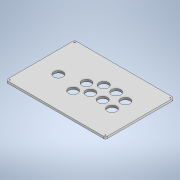
# Autodesk Inventor part: sega_straight
Saved by Autodesk Inventor 2022 (Build 260153000, 153)
## iProperties
Created: 2022-12-25
Part Number: sega_straight
Material: Generic
Document SubType Name: Modeling
Designer: Bunny
Density: 1 g/cm^3
Appearance: Default
Author: Bunny
Autodesk Inventor part; units mm, degrees
ref_plane "YZ Plane" through (0, 0, 0) normal (1, 0, 0) x (0, 1, 0)
ref_plane "XZ Plane" through (0, 0, 0) normal (0, 1, 0) x (-1, 0, 0)
ref_plane "XY Plane" through (0, 0, 0) normal (0, 0, 1) x (1, 0, 0)
sketch "Sketch1" plane through (0, 0, 0) normal (0, 1, 0) x (-1, 0, 0)
  line L0 (145, -100) -> (-145, -100)
  line L1 (-145, -100) -> (-145, 100)
  line L2 (-145, 100) -> (145, 100)
  line L3 (145, 100) -> (145, -100)
  line L4 (203, 0) -> (-203, 0) projected
  line L5 (0, -140) -> (0, 140) projected
  point P0 (0, 0)
  dimension "d30" = 290
  dimension "d31" = 200
  constraints: 8 end point, 2 parallel, 1 horizontal, 1 perpendicular, 2 other
  measures "d30" distance of L0.start L0.end
  measures "d31" distance of L0.end L1.end
extrude "Extrusion1" add sketch "Sketch1" along normal blind 6
sketch "Sketch2" plane through (0, 6, 0) normal (0, 1, 0) x (1, 0, 0)
  circle A0 centre (-19.75, -29.5) radius 13.5
  circle A1 centre (-82.75, -9.5) radius 13.5
  circle A2 centre (-19.75, 9.5) radius 13.5
  circle A3 centre (46.75, 29.5) radius 13.5
  circle A4 centre (82.75, 20.5) radius 13.5
  circle A5 centre (10.75, 29.5) radius 13.5
  circle A6 centre (10.75, -9.5) radius 13.5
  circle A7 centre (46.75, -9.5) radius 13.5
  circle A8 centre (82.75, -18.5) radius 13.5
  line L0 (-96.25, 43) -> (96.25, 43)
  line L1 (96.25, 43) -> (96.25, -43)
  line L2 (96.25, -43) -> (-96.25, -43)
  line L3 (-96.25, -43) -> (-96.25, 43)
  line L4 (145, 100) -> (-145, 100) projected
  line L5 (145, -100) -> (145, 100) projected
  line L6 (0, 140) -> (0, -140) projected
  line L7 (-203, 0) -> (203, 0) projected
  dimension "d3" = 27
  dimension "d19" = 30.5
  dimension "d20" = 36
  dimension "d23" = 19
  dimension "d24" = 9
  dimension "d25" = 36
  dimension "d26" = 11
  dimension "d27" = 9
  dimension "d28" = 11
  dimension "d29" = 63
  constraints: 9 centre point, 8 end point, 8 equal radius, 4 tangent, 4 vertical alignment, 3 horizontal alignment, 2 parallel, 1 horizontal, 1 perpendicular, 2 other
  measures "d3" diameter of A1
  measures "d19" horizontal distance of A0.centre A6.centre
  measures "d20" distance of A7.centre A6.centre
  measures "d23" vertical distance of A6.centre A2.centre
  measures "d24" vertical distance of A8.centre A6.centre
  measures "d25" horizontal distance of A8.centre A7.centre
  measures "d26" vertical distance of A0.centre A8.centre
  measures "d27" vertical distance of A4.centre A5.centre
  measures "d28" vertical distance of A2.centre A4.centre
  measures "d29" horizontal distance of A0.centre A1.centre
extrude "Extrusion2" cut sketch "Sketch2" against normal blind 10 contours A0 | A8 | L6 A6 L7 | A6 L6 | A1 L7 | A1 L7 | A4 | A3 | A6 L7 | L7 A7 | A7 L7 | L6 A5 | A5 L6 | L7 A2 | A2 L7 picked at (6.7806, -6.3333)
fillet "Fillet1" radius 5 4 edges at (-145, 3, 100) (145, 3, 100) (145, 3, -100) (-145, 3, -100)
sketch "Sketch3" plane through (0, 6, 0) normal (0, 1, 0) x (1, 0, 0)
  circle A0 centre (-139.6667, 94.6667) radius 1.5
  line L0 (140, 100) -> (-140, 100) projected
  line L1 (-145, 95) -> (-145, -95) projected
  point P0 (0, 0)
  dimension "d35" = 5.3333
  dimension "d36" = 5.3333
  dimension "d37" = 3
  constraints: 1 centre point
  measures "d35" distance from line of L0 A0.centre
  measures "d36" distance from line of L1 A0.centre
  measures "d37" diameter of A0
extrude "Extrusion3" cut sketch "Sketch3" against normal blind 10
pattern_linear "Rectangular Pattern1" count 2 spacing 279.3333 along (1, 0, 0) count 2 spacing 189.3333 along (0, 0, 1) of "Extrusion3"
equation "\"d30\" = BoxLength"
equation "\"d31\" = BoxWidth"
equation "\"d0\" = SheetThickness"
equation "\"d3\" = button_hole_outer"
equation "\"d35\" = 0.666667 * CornerOffset + 0.333333 * SheetThickness"
equation "\"d36\" = 0.666667 * CornerOffset + 0.333333 * SheetThickness"
equation "\"d42\" = BoxLength - 1.33333 * CornerOffset - 0.666667 * SheetThickness"
equation "\"d45\" = BoxWidth - 1.33333 * CornerOffset - 0.666667 * SheetThickness"
equation "\"button_hole_outer\" = 27"
equation "\"BoxLength\" = 290"
equation "\"BoxWidth\" = 200"
equation "\"SheetThickness\" = 6"
equation "\"CornerOffset\" = 5"
body "Solid1"
